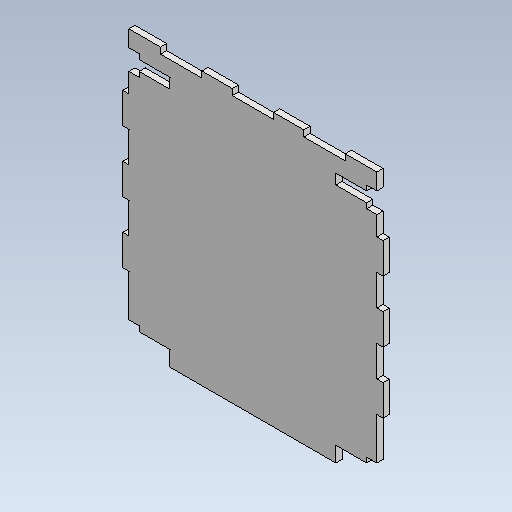
# Autodesk Inventor part: bed_acrylic_floor
Saved by Autodesk Inventor 2025 (Build 290162000, 162)
## iProperties
Created: 2025-08-24
Part Number: bed_acrylic_floor
Material: Generic
Document SubType Name: Modeling
Designer: HP
Density: 1 g/cm^3
Appearance: Default
Author: HP
Autodesk Inventor part; units mm, degrees
ref_plane "YZ Plane" through (0, 0, 0) normal (1, 0, 0) x (0, 1, 0)
ref_plane "XZ Plane" through (0, 0, 0) normal (0, 1, 0) x (-1, 0, 0)
ref_plane "XY Plane" through (0, 0, 0) normal (0, 0, 1) x (1, 0, 0)
sketch "Sketch1" plane through (0, 0, 0) normal (0, 0, 1) x (1, 0, 0)
  line L0 (-63.5, -66.5) -> (63.5, -66.5)
  line L1 (63.5, -66.5) -> (63.5, 66.5)
  line L2 (63.5, 66.5) -> (-63.5, 66.5)
  line L3 (-63.5, 66.5) -> (-63.5, -66.5)
  line L4 (-63.5, -66.5) -> (63.5, 66.5) construction
  line L5 (63.5, -66.5) -> (-63.5, 66.5) construction
  line L6 (-45.1, 66.5) -> (-24.9, 66.5)
  line L7 (-24.9, 66.5) -> (-24.9, 63.5)
  line L8 (-24.9, 63.5) -> (-45.1, 63.5)
  line L9 (-45.1, 63.5) -> (-45.1, 66.5)
  line L10 (-45.1, 66.5) -> (-24.9, 63.5) construction
  line L11 (-24.9, 66.5) -> (-45.1, 63.5) construction
  line L12 (-10.1, 66.5) -> (10.1, 66.5)
  line L13 (10.1, 66.5) -> (10.1, 63.5)
  line L14 (10.1, 63.5) -> (-10.1, 63.5)
  line L15 (-10.1, 63.5) -> (-10.1, 66.5)
  line L16 (-10.1, 66.5) -> (10.1, 63.5) construction
  line L17 (10.1, 66.5) -> (-10.1, 63.5) construction
  line L18 (24.9, 66.5) -> (45.1, 66.5)
  line L19 (45.1, 66.5) -> (45.1, 63.5)
  line L20 (45.1, 63.5) -> (24.9, 63.5)
  line L21 (24.9, 63.5) -> (24.9, 66.5)
  line L22 (24.9, 66.5) -> (45.1, 63.5) construction
  line L23 (45.1, 66.5) -> (24.9, 63.5) construction
  line L24 (-63.5, 39) -> (-60.5, 39)
  line L25 (-60.5, 39) -> (-60.5, 24) construction
  line L26 (-60.5, 24) -> (-63.5, 24)
  line L27 (-63.5, 24) -> (-63.5, 39)
  line L28 (-63.5, 39) -> (-60.5, 24) construction
  line L29 (-60.5, 39) -> (-63.5, 24) construction
  line L30 (-63.5, 9) -> (-60.5, 9)
  line L31 (-60.5, 9) -> (-60.5, -6) construction
  line L32 (-60.5, -6) -> (-63.5, -6)
  line L33 (-63.5, -6) -> (-63.5, 9)
  line L34 (-63.5, 9) -> (-60.5, -6) construction
  line L35 (-60.5, 9) -> (-63.5, -6) construction
  line L36 (-63.5, -21) -> (-60.5, -21)
  line L37 (-60.5, -21) -> (-60.5, -36) construction
  line L38 (-60.5, -36) -> (-63.5, -36)
  line L39 (-63.5, -36) -> (-63.5, -21)
  line L40 (-63.5, -21) -> (-60.5, -36) construction
  line L41 (-60.5, -21) -> (-63.5, -36) construction
  line L42 (-60.5, 39) -> (-60.5, 66.5)
  line L43 (-60.5, 24) -> (-60.5, 9)
  line L44 (-60.5, -6) -> (-60.5, -21)
  line L45 (-60.5, 51) -> (-40.5, 51)
  line L46 (-40.5, 51) -> (-40.5, 56)
  line L47 (-40.5, 56) -> (-60.5, 56)
  line L48 (-60.5, 56) -> (-60.5, 51)
  line L49 (-60.5, 51) -> (-40.5, 56) construction
  line L50 (-40.5, 51) -> (-60.5, 56) construction
  line L51 (-60.5, -64) -> (-40.5, -64)
  line L52 (-40.5, -66.5) -> (-40.5, -59)
  line L53 (-40.5, -59) -> (-60.5, -59)
  line L54 (-60.5, -59) -> (-60.5, -64)
  line L55 (-60.5, -64) -> (-40.5, -59) construction
  line L56 (-40.5, -64) -> (-60.5, -59) construction
  line L57 (-60.5, 48.5) -> (-55.5, 48.5)
  line L58 (-55.5, 48.5) -> (-55.5, 58.5)
  line L59 (-55.5, 58.5) -> (-60.5, 58.5)
  line L60 (-60.5, 58.5) -> (-60.5, 48.5)
  line L61 (-60.5, 48.5) -> (-55.5, 58.5) construction
  line L62 (-55.5, 48.5) -> (-60.5, 58.5) construction
  line L63 (-60.5, -66.5) -> (-55.5, -66.5)
  line L64 (-55.5, -66.5) -> (-55.5, -56.5)
  line L65 (-55.5, -56.5) -> (-60.5, -56.5)
  line L66 (-60.5, -56.5) -> (-60.5, -66.5)
  line L67 (-60.5, -66.5) -> (-55.5, -56.5) construction
  line L68 (-55.5, -66.5) -> (-60.5, -56.5) construction
  line L69 (-60.5, -36) -> (-60.5, -66.5)
  point P0 (0, 0)
  point P1 (-35, 65)
  point P2 (0, 65)
  point P3 (35, 65)
  point P4 (0, 66.5)
  point P5 (-62, 31.5)
  point P6 (-62, 1.5)
  point P7 (-62, -28.5)
  point P8 (45.1, 66.5)
  point P9 (24.9, 66.5)
  point P10 (10.1, 66.5)
  point P11 (-63.5, -36)
  point P12 (-63.5, -6)
  point P13 (-63.5, 9)
  point P14 (-63.5, 39)
  point P15 (-50.5, 53.5)
  point P16 (-50.5, -61.5)
  point P17 (-60.5, 56)
  point P18 (-60.5, 51)
  point P19 (-58, 53.5)
  point P20 (-40.5, 53.5)
  point P21 (-58, -61.5)
  point P22 (-55.5, 56)
  point P23 (-55.5, 51)
  point P24 (-55.5, -59)
  point P25 (-55.5, -64)
  dimension "d0" = 127
  dimension "d1" = 133
  dimension "d2" = 3
  dimension "d3" = 20.2
  dimension "d5" = 3
  dimension "d6" = 20.2
  dimension "d9" = 3
  dimension "d10" = 20.2
  dimension "d13" = 35
  dimension "d14" = 35
  dimension "d15" = 15
  dimension "d16" = 3
  dimension "d17" = 15
  dimension "d18" = 3
  dimension "d19" = 15
  dimension "d20" = 3
  dimension "d21" = 30
  dimension "d22" = 30
  dimension "d23" = 35
  dimension "d31" = 5
  dimension "d32" = 20
  dimension "d33" = 5
  dimension "d34" = 20
  dimension "d35" = 5
  dimension "d36" = 13
  dimension "d37" = 5
  dimension "d38" = 10
  dimension "d39" = 5
  dimension "d40" = 10
  constraints: 140 end point, 24 midpoint, 22 parallel, 13 perpendicular, 11 horizontal, 10 collinear, 4 point on line, 2 horizontal alignment, 1 vertical alignment
  measures "d0" distance of L2.end L1.end
  measures "d1" distance between parallel lines of L0 L2
  measures "d2" distance between parallel lines of L8 L6
  measures "d3" distance between parallel lines of L7 L9
  measures "d5" distance between parallel lines of L14 L12
  measures "d6" distance between parallel lines of L13 L15
  measures "d9" distance between parallel lines of L20 L18
  measures "d10" distance between parallel lines of L19 L21
  measures "d13" distance of point (0, 65) point (-35, 65)
  measures "d14" distance of point (35, 65) point (0, 65)
  measures "d15" distance between parallel lines of L26 L24
  measures "d16" distance between parallel lines of L25 L27
  measures "d17" distance between parallel lines of L32 L30
  measures "d18" distance between parallel lines of L31 L33
  measures "d19" distance between parallel lines of L38 L36
  measures "d20" distance between parallel lines of L37 L39
  measures "d21" distance of point (-62, 1.5) point (-62, 31.5)
  measures "d22" distance of point (-62, -28.5) point (-62, 1.5)
  measures "d23" distance from line of L2 point (-62, 31.5)
  measures "d31" distance between parallel lines of L45 L47
  measures "d32" distance between parallel lines of L46 L48
  measures "d33" distance between parallel lines of L51 L53
  measures "d34" distance between parallel lines of L52 L54
  measures "d35" distance from line of L0 point (-50.5, -61.5)
  measures "d36" distance from line of L2 point (-50.5, 53.5)
  measures "d37" distance of L59.end L58.end
  measures "d38" distance of L58.end L57.end
  measures "d39" distance between parallel lines of L64 L66
  measures "d40" distance between parallel lines of L63 L65
extrude "Extrusion1" add sketch "Sketch1" along normal blind 3 contours L3 L38 L69 L66 L54 L0 | L66 L51 L64 L0 | L3 L36 L44 L32 L30 L43 L26 L24 L42 L57 L58 L45 L46 L47 L59 L2 L9 L8 L7 L15 L14 L13 L21 L20 L19 L1 L0 L52 L53 L64 L65 L69 L38 | L64 L51 L52 L0 | L54 L53 L64 L51 | L3 L32 L44 L36 | L64 L53 L52 L51 | L66 L65 L64 L53 | L3 L26 L43 L30 | L3 L2 L42 L24 | L42 L45 L58 L57 | L59 L58 L47 L42 | L42 L47 L58 L45 | L58 L47 L46 L45
extrude "Extrusion2" cut sketch "Sketch1" along normal through all contours L3 L38 L69 L66 L54 L0 | L66 L51 L64 L0 | L64 L51 L52 L0 | L54 L53 L64 L51 | L3 L32 L44 L36 | L64 L53 L52 L51 | L66 L65 L64 L53 | L3 L26 L43 L30 | L3 L2 L42 L24 | L42 L45 L58 L57 | L59 L58 L47 L42 | L42 L47 L58 L45 | L58 L47 L46 L45
mirror "Mirror1" about plane through (0, 0, 0) normal (1, 0, 0) of "Extrusion2"
equation "\"d5\" = d2"
equation "\"d6\" = d3"
equation "\"d9\" = d2"
equation "\"d10\" = d11"
equation "\"d14\" = d13"
equation "\"d16\" = d2"
equation "\"d17\" = d15"
equation "\"d18\" = d16"
equation "\"d19\" = d17"
equation "\"d20\" = d18"
equation "\"d22\" = d21"
equation "\"d33\" = d31"
equation "\"d34\" = d32"
equation "\"d11\" = 20.2"
body "Solid1"
